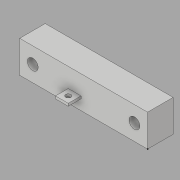
# Autodesk Inventor part: g_griper side
Saved by Autodesk Inventor 2019 (Build 230136000, 136)
## iProperties
Created: 2021-10-30
Part Number: g_griper side
Material: Generic
Document SubType Name: Modeling
Designer: Mohamed
Density: 1 g/cm^3
Appearance: Default
Author: Mohamed
Autodesk Inventor part; units mm, degrees
ref_plane "YZ Plane" through (0, 0, 0) normal (1, 0, 0) x (0, 1, 0)
ref_plane "XZ Plane" through (0, 0, 0) normal (0, 1, 0) x (-1, 0, 0)
ref_plane "XY Plane" through (0, 0, 0) normal (0, 0, 1) x (1, 0, 0)
sketch "Sketch1" plane through (0, 0, 0) normal (0, 1, 0) x (-1, 0, 0)
  line L0 (0, 0) -> (100, 0)
  line L1 (100, 0) -> (100, -20)
  line L2 (100, -20) -> (0, -20)
  line L3 (0, -20) -> (0, 0)
  dimension "d0" = 100
  dimension "d1" = 20
  constraints: 8 end point, 3 perpendicular, 1 horizontal
  measures "d0" distance of L0.start L0.end
  measures "d1" distance of L0.end L1.end
extrude "Extrusion1" add sketch "Sketch1" along normal blind 25
sketch "Sketch2" plane through (-100, 0, 0) normal (0, 0, 1) x (1, 0, 0)
  point P0 (100, 0)
sketch "Sketch3" plane through (-100, 0, 0) normal (0, 0, 1) x (1, 0, 0)
  line L0 (0, 25) -> (100, 25) projected
  circle A0 centre (10.25, 12.5) radius 4.25
  circle A1 centre (89.75, 12.5) radius 4.25
  point P0 (100, 0)
  dimension "d7" = 8.5
  dimension "d8" = 8.5
  constraints: 2 centre point
  measures "d7" diameter of A0
  measures "d8" diameter of A1
extrude "Extrusion2" cut sketch "Sketch3" against normal blind 20
sketch "Sketch4" plane through (-100, 0, 0) normal (0, 0, 1) x (1, 0, 0)
  point P0 (100, 0)
sketch "Sketch5" plane through (-100, 0, 0) normal (0, 0, 1) x (1, 0, 0)
  line L0 (100, 25) -> (0, 25) projected
  line L1 (0, 25) -> (100, 25) projected
  line L2 (43, 8) -> (48, 8)
  line L3 (48, 8) -> (38, 8)
  line L4 (38, 8) -> (38, 10)
  line L5 (38, 10) -> (48, 10)
  line L6 (48, 10) -> (48, 8)
  point P0 (100, 0)
  dimension "d27" = 5
  dimension "d30" = 10
  constraints: 10 end point, 2 perpendicular, 1 horizontal
  measures "d27" distance of L2.start L2.end
  measures "d30" distance of L4.end L5.end
extrude "Extrusion3" add sketch "Sketch5" along normal blind 10
sketch "Sketch6" plane through (-62, 18, 0) normal (0, 1, 0) x (1, 0, 0)
  line L0 (10, -10) -> (0, -10) projected
  circle A0 centre (5, -5) radius 2
  point P0 (62, 0)
  dimension "d22" = 4
  constraints: 1 centre point
  measures "d22" diameter of A0
extrude "Extrusion4" [suppressed]
sketch "Sketch7" plane through (-62, 10, 0) normal (0, 1, 0) x (1, 0, 0)
  line L0 (0, -10) -> (10, -10) projected
  circle A0 centre (5, -5) radius 2
  point P0 (62, 0)
  dimension "d32" = 4
  constraints: 1 centre point
  measures "d32" diameter of A0
extrude "Extrusion5" cut sketch "Sketch7" against normal blind 2
body "Solid1"
